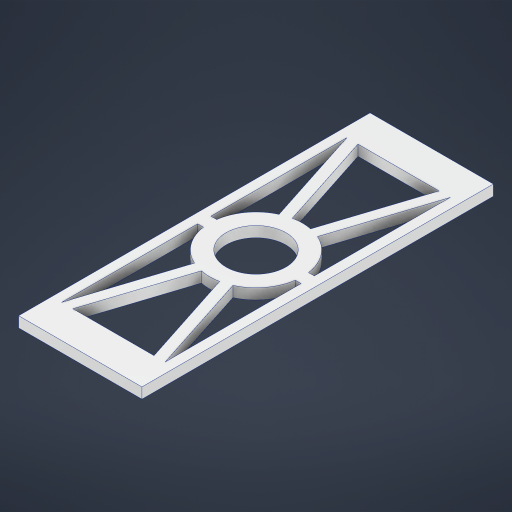
# Autodesk Inventor part: A_AxisKrovatka
Saved by Autodesk Inventor 2024 (Build 280153000, 153)
## iProperties
Created: 2023-12-22
Part Number: A_AxisKrovatka
Material: Aluminum 6061
Document SubType Name: Modeling
Designer: KirikDK
Mass: 2197.01 g
Surface Area: 1721.41 cm^2
Volume: 813.706 cm^3
Density: 2.7 g/cm^3
Appearance: Aluminum - Flat
Author: KirikDK
Autodesk Inventor part; units mm, degrees
ref_plane "YZ Plane" through (0, 0, 0) normal (1, 0, 0) x (0, 1, 0)
ref_plane "XZ Plane" through (0, 0, 0) normal (0, 1, 0) x (-1, 0, 0)
ref_plane "XY Plane" through (0, 0, 0) normal (0, 0, 1) x (1, 0, 0)
sketch "Sketch1" plane through (0, 0, 0) normal (0, 1, 0) x (-1, 0, 0)
  line L0 (15.3, 271) -> (-170.7, 271)
  line L1 (-170.7, 271) -> (-170.7, -271)
  line L2 (-170.7, -271) -> (15.3, -271)
  line L3 (15.3, -271) -> (15.3, 271)
  line L4 (-77.7, 271) -> (-77.7, -271)
  line L5 (-170.7, 0) -> (15.3, 0)
  circle A0 centre (-77.7, 0) radius 45
  point P0 (0, 0)
  dimension "d0" = 542
  dimension "d1" = 186
  dimension "d2" = 90
  constraints: 12 end point, 5 midpoint, 2 parallel, 1 centre point, 1 horizontal, 1 perpendicular
  measures "d0" distance of L2.end L0.start
  measures "d1" distance of L0.start L0.end
  measures "d2" diameter of A0
extrude "Extrusion1" add sketch "Sketch1" along normal blind 16 contours L3 L5 A0 L4 L0 | L4 A0 L5 L1 L0 | L3 L2 L4 A0 L5 | L5 A0 L4 L2 L1
sketch "Sketch2" plane through (170.7, 0, 271) normal (1, 0, 0) x (0, 0, -1)
  line L0 (0, 0) -> (0, 16) projected
  line L1 (0, 6) -> (-25, 6)
  line L2 (-25, 6) -> (-25, 0)
  line L3 (-25, 0) -> (0, 0)
  line L4 (0, 0) -> (0, 6)
  line L5 (542, 0) -> (542, 16) projected
  line L6 (542, 6) -> (567, 6)
  line L7 (567, 6) -> (567, 0)
  line L8 (567, 0) -> (542, 0)
  line L9 (542, 0) -> (542, 6)
  line L10 (542, 16) -> (527, 16)
  line L11 (527, 16) -> (527, 66)
  line L12 (527, 66) -> (542, 66)
  line L13 (542, 66) -> (542, 16)
  line L14 (0, 16) -> (15, 16)
  line L15 (15, 16) -> (15, 66)
  line L16 (15, 66) -> (0, 66)
  line L17 (0, 66) -> (0, 16)
  point P0 (271, 0)
  dimension "d5" = 6
  dimension "d6" = 25
  dimension "d7" = 25
  dimension "d8" = 50
  dimension "d9" = 15
  dimension "d10" = 15
  dimension "d11" = 50
  constraints: 32 end point, 8 parallel, 4 horizontal, 4 perpendicular, 3 point on line
  measures "d5" distance of L6.end L7.end
  measures "d6" distance of L7.end L8.end
  measures "d7" distance of L2.end L3.end
  measures "d8" distance of L12.end L5.end
  measures "d9" distance of L11.end L12.end
  measures "d10" distance of L15.end L16.end
  measures "d11" distance of L14.end L15.end
extrude "Extrusion2" add sketch "Sketch2" against normal up to surface (186 mm away)
sketch "Sketch3" plane through (0, 16, 0) normal (0, 1, 0) x (1, 0, 0)
  line L0 (170.7, 256) -> (-15.3, 256) projected
  line L1 (-15.3, 256) -> (-15.3, -256) projected
  line L2 (-15.3, -256) -> (170.7, -256) projected
  line L3 (170.7, -256) -> (170.7, 256) projected
  circle A0 centre (77.7, 0) radius 45 projected
  line L4 (-0.3, -241) -> (-0.3, 241)
  line L5 (-0.3, 241) -> (155.7, 241)
  line L6 (155.7, 241) -> (155.7, -241)
  line L7 (155.7, -241) -> (-0.3, -241)
  circle A1 centre (77.7, 0) radius 70
  line L8 (155.7, -241) -> (-0.3, 241)
  line L9 (155.7, 241) -> (-0.3, -241)
  line L10 (148.0887, 243.4634) -> (-7.9113, -238.5366)
  line L11 (163.3113, 238.5366) -> (7.3113, -243.4634)
  line L12 (148.0887, -243.4634) -> (-7.9113, 238.5366)
  line L13 (163.3113, -238.5366) -> (7.3113, 243.4634)
  line L14 (-0.3, -10) -> (155.7, -10)
  line L15 (155.7, -10) -> (155.7, 10)
  line L16 (155.7, 10) -> (-0.3, 10)
  line L17 (-0.3, 10) -> (-0.3, -10)
  point P0 (0, 0)
  point P1 (77.7, 0)
  point P2 (77.7, 0)
  point P3 (146.982, 10)
  point P4 (155.7, 215.0197)
  point P5 (106.7248, 63.699)
  point P6 (146.982, -10)
  point P7 (106.7248, -63.699)
  point P8 (155.7, -215.0197)
  point P9 (8.1086, 241)
  point P10 (63.8977, 68.6258)
  point P11 (91.5023, 68.6258)
  point P12 (147.2914, 241)
  point P13 (-0.3, 10)
  point P14 (8.418, 10)
  point P15 (48.6752, 63.699)
  point P16 (-0.3, 215.0197)
  point P17 (8.418, -10)
  point P18 (-0.3, -215.0197)
  point P19 (48.6752, -63.699)
  point P20 (147.2914, -241)
  point P21 (91.5023, -68.6258)
  point P22 (63.8977, -68.6258)
  point P23 (8.1086, -241)
  dimension "d14" = 25
  dimension "d15" = 15
  dimension "d16" = 10
  dimension "d17" = 10
  dimension "d18" = 8
  dimension "d19" = 8
  dimension "d20" = 8
  dimension "d21" = 8
  constraints: 28 end point, 6 parallel, 2 midpoint, 2 point on line, 1 centre point, 1 horizontal, 1 perpendicular, 3 other
  measures "d14" radial gap between concentric circles of A0 A1
  measures "d15" distance between parallel lines of L1 L4
  measures "d16" distance from line of L16 point (77.7, 0)
  measures "d17" distance from line of L14 point (77.7, 0)
  measures "d18" distance between parallel lines of L12 L8
  measures "d19" distance between parallel lines of L8 L13
  measures "d20" distance between parallel lines of L9 L10
  measures "d21" distance between parallel lines of L9 L11
extrude "Extrusion3" cut sketch "Sketch3" against normal blind 20 contours A1 L11 L6 L16 | L14 L6 L13 A1 | A1 L13 L5 L10 | L12 L7 L11 A1 | A1 L16 L4 L12 | L10 L4 L14 A1
sketch "Sketch4" plane through (0, 16, 0) normal (0, 1, 0) x (1, 0, 0)
  line L0 (-0.3, 10) -> (-0.3, 215.0197) projected
  line L1 (-0.3, 215.0197) -> (156, 215.0197)
  line L2 (156, 215.0197) -> (156, 245)
  line L3 (156, 245) -> (-0.3, 245)
  line L4 (-0.3, 245) -> (-0.3, 215.0197)
  line L5 (-0.3, -215.0197) -> (48.6752, -63.699) projected
  line L6 (-0.3, -215.0197) -> (158, -215.0197)
  line L7 (158, -215.0197) -> (158, -245)
  line L8 (158, -245) -> (-0.3, -245)
  line L9 (-0.3, -245) -> (-0.3, -215.0197)
  point P0 (0, 0)
  constraints: 16 end point, 4 parallel, 2 horizontal, 2 perpendicular
extrude "Extrusion4" add sketch "Sketch4" against normal up to surface (16 mm away)
sketch "Sketch5" plane through (0, 16, 0) normal (0, 1, 0) x (1, 0, 0)
  line L0 (-72, -376) -> (216, -376)
  line L1 (216, -376) -> (216, -255.0197)
  line L2 (216, -255.0197) -> (-72, -255.0197)
  line L3 (-72, -255.0197) -> (-72, -376)
  line L4 (-67, 399) -> (218, 399)
  line L5 (218, 399) -> (218, 255.0197)
  line L6 (218, 255.0197) -> (-67, 255.0197)
  line L7 (-67, 255.0197) -> (-67, 399)
  line L8 (16.5171, 215.0197) -> (138.8829, 215.0197) projected
  line L9 (138.8829, -215.0197) -> (16.5171, -215.0197) projected
  point P0 (0, 0)
  dimension "d26" = 40
  dimension "d27" = 40
  constraints: 16 end point, 4 parallel, 2 horizontal, 2 perpendicular
  measures "d26" distance between parallel lines of L6 L8
  measures "d27" distance between parallel lines of L9 L2
extrude "Extrusion5" cut sketch "Sketch5" along normal mid plane 100
sketch "Sketch6" plane through (0, 16, 0) normal (0, 1, 0) x (1, 0, 0)
  line L0 (-15.3, 255.0197) -> (-15.3, -255.0197) projected
  line L1 (-15.3, 255.0197) -> (170.7, 255.0197)
  line L2 (170.7, 255.0197) -> (170.7, 265.0197)
  line L3 (170.7, 265.0197) -> (-15.3, 265.0197)
  line L4 (-15.3, 265.0197) -> (-15.3, 255.0197)
  line L5 (-15.3, -255.0197) -> (170.7, -255.0197)
  line L6 (170.7, -255.0197) -> (170.7, -265.0197)
  line L7 (170.7, -265.0197) -> (-15.3, -265.0197)
  line L8 (-15.3, -265.0197) -> (-15.3, -255.0197)
  line L9 (-15.3, -255.0197) -> (170.7, -255.0197) projected
  point P0 (0, 0)
  dimension "d30" = 10
  dimension "d31" = 0
  dimension "d32" = 10
  constraints: 16 end point, 4 parallel, 2 horizontal, 2 perpendicular, 2 point on line
  measures "d30" distance between parallel lines of L5 L7
  measures "d31" distance between parallel lines of L9 L5
  measures "d32" distance between parallel lines of L1 L3
extrude "Extrusion6" add sketch "Sketch6" against normal up to surface (16 mm away)
body "Solid1"
